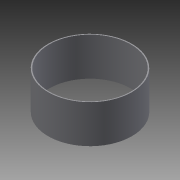
# Autodesk Inventor part: curved piece
Saved by Autodesk Inventor 2015 (Build 190159000, 159)
## iProperties
Created: 2014-10-04
Part Number: curved piece
Material: Generic
Document SubType Name: Modeling
Designer: jesse
Density: 1 g/cm^3
Appearance: Default
Author: jesse
Autodesk Inventor part; units mm, degrees
ref_plane "YZ Plane" through (0, 0, 0) normal (1, 0, 0) x (0, 1, 0)
ref_plane "XZ Plane" through (0, 0, 0) normal (0, 1, 0) x (-1, 0, 0)
ref_plane "XY Plane" through (0, 0, 0) normal (0, 0, 1) x (1, 0, 0)
sketch "Sketch1" plane through (0, 0, 0) normal (0, 1, 0) x (-1, 0, 0)
  arc A0 (-95.25, 0) -> (0, -95.25) centre (0, 0) ccw
  arc A1 (-97.65, 0) -> (0, -97.65) centre (0, 0) ccw
  line L0 (0, -37.9954) -> (0, -112.7989)
  line L1 (-62.3225, 0) -> (-123.319, 0)
  dimension "d0" = 190.5
  dimension "d1" = 2.4
  constraints: 4 end point, 4 point on circle, 4 point on line, 2 centre point, 1 coincident, 1 horizontal, 1 vertical
  measures "d0" diameter of A0
  measures "d1" radial gap between concentric circles of A0 A1
extrude "Extrusion2" add sketch "Sketch1" along normal blind 88.9
body "Solid2"
